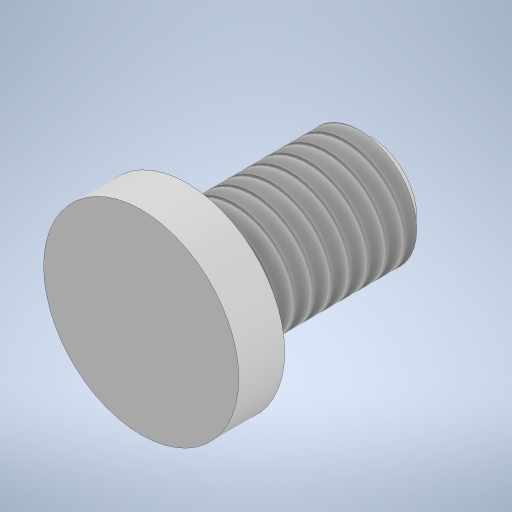
# Autodesk Inventor part: Болт штурвал
Saved by Autodesk Inventor 2023 (Build 270158000, 158)
## iProperties
Created: 2022-05-01
Part Number: Болт штурвал
Material: Типовые
Document SubType Name: Modeling
Designer: User
Density: 1 g/cm^3
Appearance: По умолчанию
Author: User
Autodesk Inventor part; units mm, degrees
ref_plane "YZ Plane" through (0, 0, 0) normal (1, 0, 0) x (0, 1, 0)
ref_plane "XZ Plane" through (0, 0, 0) normal (0, 1, 0) x (-1, 0, 0)
ref_plane "XY Plane" through (0, 0, 0) normal (0, 0, 1) x (1, 0, 0)
sketch "Эскиз1" plane through (0, 0, 0) normal (0, 1, 0) x (-1, 0, 0)
  line L0 (0, 0) -> (4.25, 0)
  line L1 (4.25, 0) -> (4.25, -2)
  line L2 (0, -2) -> (2.5, -2)
  line L3 (2.5, -2.6792) -> (2.5, -10)
  line L4 (2.5, -10) -> (0, -10)
  line L5 (0, -10) -> (0, -2)
  line L6 (2.5, -2) -> (3, -2)
  line L7 (3, -2) -> (3, -2.6792)
  line L8 (3, -2.6792) -> (2.5, -2.6792)
  line L9 (3, -2) -> (4.25, -2)
  line L10 (0, 0) -> (0, -2)
  dimension "d0" = 4.25
  dimension "d1" = 2
  dimension "d3" = 8
  dimension "d4" = 0.5
  constraints: 22 end point, 6 perpendicular, 2 horizontal, 1 parallel, 1 point on line, 1 vertical
  measures "d0" distance of L0.start L0.end
  measures "d1" distance of L0.end L1.end
  measures "d3" distance of L2.end L3.end
  measures "d4" distance of L2.end L6.end
revolve "Вращение1" add sketch "Эскиз1" angle 360 about axis through (0, 0, -10) along (0, 0, 1)
thread "Резьба1" size "M5x0.8" class "6g" standard "ISO Metric profile" full length
chamfer "Фаска1" distance 0.5 angle 45 1 edges at (2.5, 0, -10)
